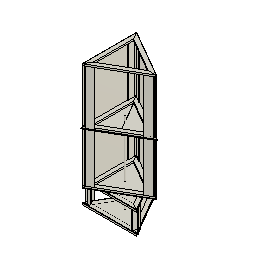
Periaktos (Autodesk Fusion 360 design; units mm, degrees)
Autodesk Fusion 360 part; units mm, degrees
sketch "Triangle" plane through (0, 0, 0) normal (0, 0, 1) x (1, 0, 0)
  line L0 (-609.6, -351.9527) -> (-609.6, -356.9527)
  line L1 (455.6207, -263.0527) -> (0, 526.1054)
  line L2 (0, 703.9054) -> (0, 526.1054)
  line L3 (0, -351.9527) -> (0, 703.9054)
  line L4 (-609.6, -351.9527) -> (-613.9301, -349.4527)
  line L5 (0, 703.9054) -> (-4.3301, 706.4054)
  line L6 (609.6, -351.9527) -> (613.9301, -349.4527)
  line L7 (0, 703.9054) -> (4.3301, 706.4054)
  line L8 (455.6207, -263.0527) -> (0, 0) construction
  circle A0 centre (0, 0) radius 11.1125
  line L9 (-609.6, -351.9527) -> (-455.6207, -263.0527)
  line L10 (609.6, -351.9527) -> (0, 703.9054)
  line L11 (0, 526.1054) -> (0, 0) construction
  line L12 (613.9301, -349.4527) -> (4.3301, 706.4054)
  line L13 (-609.6, -351.9527) -> (609.6, -351.9527)
  line L14 (-455.6207, -263.0527) -> (455.6207, -263.0527)
  line L15 (-4.3301, 706.4054) -> (-613.9301, -349.4527)
  line L16 (-609.6, -356.9527) -> (609.6, -356.9527)
  line L17 (609.6, -351.9527) -> (455.6207, -263.0527)
  line L18 (609.6, -351.9527) -> (609.6, -356.9527)
  line L19 (0, 703.9054) -> (-609.6, -351.9527)
  line L20 (-455.6207, -263.0527) -> (0, 0) construction
  line L21 (0, 526.1054) -> (-455.6207, -263.0527)
  line L22 (-609.6, -351.9527) -> (-558.8, -351.9527) construction
  point P0 (0, -263.0527)
  dimension "d82" = 88.9
  dimension "d83" = 88.9
  dimension "d84" = 88.9
  dimension "d85" = 5
  dimension "d86" = 5
  dimension "d87" = 5
  dimension "d88" = 1219.2
  dimension "d89" = 22.225
  dimension "d108" = 50.8
  constraint perpendicular L5 L15
  constraint perpendicular L7 L12
  constraint perpendicular L0 L16
  constraint perpendicular L4 L15
  constraint perpendicular L6 L12
  constraint perpendicular L16 L18
  constraint horizontal L13
  constraint coincident L8.end A0.centre
  constraint equal L13 L19
  constraint equal L10 L13
  constraint equal L11 L20
  constraint equal L8 L11
  constraint midpoint L3.start L13
  constraint perpendicular L0 L22
  constraint midpoint L14 P0
  measures "d82" distance of L1 L10
  measures "d83" distance of L19 L21
  measures "d84" distance of L13 L14
  measures "d85" distance of L10 L12
  measures "d86" distance of L15 L19
  measures "d87" distance of L13 L16
  measures "d88" distance of L0.start L6.start
  measures "d89" diameter of A0
  measures "d108" distance of L0.start L22.end
sketch "Supports" plane through (0, 0, 0) normal (0, 0, 1) x (1, 0, 0) in component "Periaktos"
  line L0 (-609.6, -351.9527) -> (609.6, -351.9527) construction
  line L1 (0, 703.9054) -> (-609.6, -351.9527) construction
  line L2 (609.6, -351.9527) -> (0, 703.9054) construction
  line L3 (-558.8, -351.9527) -> (-406.4, -351.9527)
  line L4 (-406.4, -351.9527) -> (-406.4, -339.2527)
  line L5 (-406.4, -339.2527) -> (-558.8, -339.2527)
  line L6 (-558.8, -339.2527) -> (-558.8, -351.9527)
  line L7 (-609.6, -351.9527) -> (-584.2, -307.9586) construction
  line L8 (-584.2, -307.9586) -> (-573.2015, -314.3086)
  line L9 (-573.2015, -314.3086) -> (-497.0015, -182.3264)
  line L10 (-497.0015, -182.3264) -> (-508, -175.9764)
  line L11 (-508, -175.9764) -> (-584.2, -307.9586)
  line L12 (-609.6, -351.9527) -> (-558.8, -351.9527) construction
  line L13 (584.2, -307.9586) -> (508, -175.9764)
  line L14 (573.2015, -314.3086) -> (584.2, -307.9586)
  line L15 (497.0015, -182.3264) -> (573.2015, -314.3086)
  line L16 (508, -175.9764) -> (497.0015, -182.3264)
  line L17 (406.4, -351.9527) -> (558.8, -351.9527)
  line L18 (406.4, -339.2527) -> (406.4, -351.9527)
  line L19 (558.8, -339.2527) -> (406.4, -339.2527)
  line L20 (558.8, -351.9527) -> (558.8, -339.2527)
  line L21 (-25.4, 659.9114) -> (-101.6, 527.9291)
  line L22 (-14.4015, 653.5614) -> (-25.4, 659.9114)
  line L23 (-90.6015, 521.5791) -> (-14.4015, 653.5614)
  line L24 (-101.6, 527.9291) -> (-90.6015, 521.5791)
  line L25 (101.6, 527.9291) -> (25.4, 659.9114)
  line L26 (90.6015, 521.5791) -> (101.6, 527.9291)
  line L27 (14.4015, 653.5614) -> (90.6015, 521.5791)
  line L28 (25.4, 659.9114) -> (14.4015, 653.5614)
  dimension "d110" = 152.4
  dimension "d111" = 12.7
  dimension "d112" = 50.8
  dimension "d113" = 12.7
  dimension "d114" = 152.4
  dimension "d115" = 50.8
  dimension "d117" = 360
  constraint coincident L0.start L1.end
  constraint parallel L1 L7
  constraint perpendicular L8 L11
  constraint perpendicular L10 L11
  constraint parallel L9 L11
  constraint collinear L1 L11
  constraint collinear L0 L3
  constraint parallel L3 L5
  constraint perpendicular L3 L6
  constraint perpendicular L3 L4
  constraint perpendicular L6 L12
  measures "d110" distance of L3.start L3.end
  measures "d111" distance of L3.start L5.end
  measures "d112" distance of L0.start L7.end
  measures "d113" distance of L7.end L8.end
  measures "d114" distance of L7.end L10.end
  measures "d115" distance of L3.start L0.start
extrude "Extrude1" add sketch "Triangle" along normal blind 12.7 from surface at 622.3 contours L2 L3 L9 L19 L21 | L3 L9 L13 L14 | L3 A0 L14 L21 | L3 L13 L14 L17 | L1 L2 L3 L10 L17 | L1 L3 A0 L14 makes body 1 in component "Periaktos"
extrude "Extrude2" add sketch "Triangle" along normal blind 38.1 from surface at 635 separate body contours L3 L9 L13 L14 | L3 L13 L14 L17 makes body 2 in component "Periaktos"
extrude "Extrude3" add sketch "Triangle" along normal blind 38.1 from surface at 635 separate body contours L2 L3 L9 L19 L21 makes body 3 in component "Periaktos"
extrude "Extrude4" add sketch "Triangle" along normal blind 38.1 from surface at 635 separate body contours L1 L2 L3 L10 L17 makes body 4 in component "Periaktos"
move_face "OffsetFaces1" offset -1.5875 4 faces at (-406.4, -351.9527, 626.5333) (203.2, -351.9527, 626.5333) (-203.2, 351.9527, 630.7667) (203.2, 351.9527, 626.5333) on bodies 1 in component "Periaktos"
extrude "Extrude5" add sketch "Triangle" against normal blind 38.1 from surface at 1841.5 separate body contours L3 L9 L13 L14 | L3 L13 L14 L17 makes body 5 in component "Periaktos"
extrude "Extrude6" add sketch "Triangle" against normal blind 38.1 from surface at 1841.5 separate body contours L2 L3 L9 L19 L21 makes body 6 in component "Periaktos"
extrude "Extrude7" add sketch "Triangle" against normal blind 38.1 from surface at 1841.5 separate body contours L1 L2 L3 L10 L17 makes body 7 in component "Periaktos"
extrude "Extrude8" add sketch "Triangle" against normal blind 12.7 from surface at 1803.4 separate body contours L2 L3 L9 L19 L21 | L3 L9 L13 L14 | L3 A0 L14 L21 makes body 8 in component "Periaktos"
extrude "Extrude9" add sketch "Triangle" against normal blind 12.7 from surface at 1803.4 separate body contours L3 L13 L14 L17 | L1 L2 L3 L10 L17 | L1 L3 A0 L14 makes body 9 in component "Periaktos"
move_face "OffsetFaces2" offset 12.7 4 faces at (-406.4, -351.9527, 1799.1667) (-203.2, 351.9527, 1794.9333) (203.2, -351.9527, 1799.1667) (203.2, 351.9527, 1799.1667) on bodies 8 9 in component "Periaktos"
extrude "Extrude10" add sketch "Triangle" against normal blind 38.1 from surface at 3060.7 separate body contours L3 L9 L13 L14 | L3 L13 L14 L17 makes body 10 in component "Periaktos"
extrude "Extrude11" add sketch "Triangle" against normal blind 38.1 from surface at 3060.7 separate body contours L2 L3 L9 L19 L21 makes body 11 in component "Periaktos"
extrude "Extrude12" add sketch "Triangle" against normal blind 38.1 from surface at 3060.7 separate body contours L1 L2 L3 L10 L17 makes body 12 in component "Periaktos"
extrude "Extrude 13" cut sketch "Supports" along normal up to surface (2349.5 mm away) from surface at 673.1 contours L3 L4 L5 L6 | L17 L18 L19 L20 bodies 5 8 9 in component "Periaktos"
extrude "Extrude14" add sketch "Supports" along normal up to surface (2349.5 mm away) from surface at 673.1 separate body contours L3 L4 L5 L6 | L17 L18 L19 L20 makes body 13 at (-508, -351.9527, 1456.2667) makes body 14 at (508, -339.2527, 1456.2667) in component "Periaktos"
extrude "Extrude15" cut sketch "Supports" along normal up to surface (2349.5 mm away) from surface at 673.1 contours L8 L9 L10 L11 | L21 L22 L23 L24 bodies 6 8 in component "Periaktos"
extrude "Extrude16" add sketch "Supports" along normal up to surface (2349.5 mm away) from surface at 673.1 separate body contours L8 L9 L10 L11 | L21 L22 L23 L24 makes body 15 at (-50.8, 615.9173, 1456.2667) makes body 16 at (-533.4, -219.9705, 1456.2667) in component "Periaktos"
extrude "Extrude17" cut sketch "Supports" along normal up to surface (2349.5 mm away) from surface at 673.1 contours L13 L14 L15 L16 | L25 L26 L27 L28 bodies 7 9 in component "Periaktos"
extrude "Extrude18" add sketch "Supports" along normal up to surface (2349.5 mm away) from surface at 673.1 separate body contours L13 L14 L15 L16 | L25 L26 L27 L28 makes body 17 at (558.8, -263.9645, 1456.2667) makes body 18 at (39.8015, 609.5673, 1456.2667) in component "Periaktos"
extrude "Extrude19" add sketch "Triangle" along normal up to surface (2438.4 mm away) from surface at 622.3 separate body contours L0 L13 L16 L18 makes body 19 in component "Periaktos"
extrude "Extrude20" add sketch "Triangle" along normal up to surface (2438.4 mm away) from surface at 622.3 separate body contours L4 L5 L15 L19 makes body 20 in component "Periaktos"
extrude "Extrude21" add sketch "Triangle" along normal up to surface (2438.4 mm away) from surface at 622.3 separate body contours L6 L7 L10 L12 makes body 21 in component "Periaktos"
sketch "Supports (2)" plane through (0, 0, 0) normal (0, 0, 1) x (1, 0, 0) in component "Pedestal"
  line L0 (-455.6207, -263.0527) -> (455.6207, -263.0527) construction
  line L1 (0, 526.1054) -> (-455.6207, -263.0527) construction
  line L2 (455.6207, -263.0527) -> (0, 526.1054) construction
  line L3 (-609.6, -351.9527) -> (609.6, -351.9527) construction
  line L4 (0, 703.9054) -> (-609.6, -351.9527) construction
  line L5 (609.6, -351.9527) -> (0, 703.9054) construction
  line L6 (-609.6, -351.9527) -> (-455.6207, -263.0527) construction
  line L7 (0, 703.9054) -> (0, 526.1054) construction
  line L8 (609.6, -351.9527) -> (455.6207, -263.0527) construction
  circle A0 centre (0, 0) radius 10.668
  line L9 (-609.6, -351.9527) -> (-584.2, -307.9586) construction
  line L10 (-584.2, -307.9586) -> (-508, -175.9764)
  line L11 (-508, -175.9764) -> (-518.9985, -169.6264)
  line L12 (-518.9985, -169.6264) -> (-595.1985, -301.6086)
  line L13 (-595.1985, -301.6086) -> (-584.2, -307.9586)
  line L14 (0, 703.9054) -> (-25.4, 659.9114) construction
  line L15 (-25.4, 659.9114) -> (-36.3985, 666.2614)
  line L16 (-36.3985, 666.2614) -> (-112.5985, 534.2791)
  line L17 (-112.5985, 534.2791) -> (-101.6, 527.9291)
  line L18 (-101.6, 527.9291) -> (-25.4, 659.9114)
  line L19 (25.4, 659.9114) -> (101.6, 527.9291)
  line L20 (36.3985, 666.2614) -> (25.4, 659.9114)
  line L21 (112.5985, 534.2791) -> (36.3985, 666.2614)
  line L22 (101.6, 527.9291) -> (112.5985, 534.2791)
  line L23 (508, -175.9764) -> (584.2, -307.9586)
  line L24 (518.9985, -169.6264) -> (508, -175.9764)
  line L25 (595.1985, -301.6086) -> (518.9985, -169.6264)
  line L26 (584.2, -307.9586) -> (595.1985, -301.6086)
  line L27 (-44.45, 602.3054) -> (44.45, 602.3054)
  line L28 (44.45, 602.3054) -> (44.45, 564.2054)
  line L29 (44.45, 564.2054) -> (-44.45, 564.2054)
  line L30 (-44.45, 564.2054) -> (-44.45, 602.3054)
  line L31 (0, 703.9054) -> (0, 602.3054) construction
  line L32 (-510.8413, -243.6079) -> (-466.3913, -320.5976)
  line L33 (-466.3913, -320.5976) -> (-499.3868, -339.6476)
  line L34 (-499.3868, -339.6476) -> (-543.8368, -262.6579)
  line L35 (-543.8368, -262.6579) -> (-510.8413, -243.6079)
  line L36 (466.3913, -320.5976) -> (510.8413, -243.6079)
  line L37 (510.8413, -243.6079) -> (543.8368, -262.6579)
  line L38 (543.8368, -262.6579) -> (499.3868, -339.6476)
  line L39 (499.3868, -339.6476) -> (466.3913, -320.5976)
  dimension "d156" = 21.336
  dimension "d157" = 50.8
  dimension "d158" = 152.4
  dimension "d159" = 12.7
  dimension "d162" = 50.8
  dimension "d163" = 12.7
  dimension "d164" = 152.4
  dimension "d168" = 360
  dimension "d181" = 88.9
  dimension "d182" = 38.1
  dimension "d183" = 101.6
  dimension "d185" = 360
  constraint coincident A0.centre origin
  constraint coincident L3.start L4.end
  constraint coincident L4 L9.end
  constraint perpendicular L10 L13
  constraint perpendicular L10 L11
  constraint parallel L10 L12
  constraint collinear L4 L10
  constraint coincident L4.start L5.end
  constraint parallel L4 L14
  constraint perpendicular L15 L18
  constraint perpendicular L17 L18
  constraint parallel L16 L18
  constraint collinear L4 L18
  constraint horizontal L27
  constraint vertical L28
  constraint horizontal L29
  constraint vertical L30
  constraint midpoint L27 L31.end
  constraint vertical L31
  measures "d156" diameter of A0
  measures "d157" distance of L3.start L9.end
  measures "d158" distance of L9.end L10.end
  measures "d159" distance of L9.end L12.end
  measures "d162" distance of L4.start L14.end
  measures "d163" distance of L14.end L15.end
  measures "d164" distance of L14.end L17.end
  measures "d181" distance of L27.start L27.end
  measures "d182" distance of L27.start L29.end
  measures "d183" distance of L4.start L31.end
extrude "Extrude1'" add sketch "Triangle" along normal blind 38.1 from surface at 38.1 separate body contours L3 L9 L13 L14 | L3 L13 L14 L17 makes body 22 in component "Pedestal"
extrude "Extrude2'" add sketch "Triangle" along normal blind 38.1 from surface at 38.1 separate body contours L2 L3 L9 L19 L21 makes body 23 in component "Pedestal"
extrude "Extrude3'" add sketch "Triangle" along normal blind 38.1 from surface at 38.1 separate body contours L1 L2 L3 L10 L17 makes body 24 in component "Pedestal"
extrude "Extrude4'" add sketch "Triangle" along normal blind 12.7 from surface at 76.2 separate body contours L2 L3 L9 L19 L21 | L3 L9 L13 L14 | L3 A0 L14 L21 | L3 L13 L14 L17 | L1 L2 L3 L10 L17 | L1 L3 A0 L14 | L3 A0 | L3 A0 makes body 25 in component "Pedestal"
extrude "Extrude5'" add sketch "Triangle" against normal blind 12.7 from surface at 558.8 separate body contours L2 L3 L9 L19 L21 | L3 L9 L13 L14 | L3 A0 L14 L21 | L3 L13 L14 L17 | L1 L2 L3 L10 L17 | L1 L3 A0 L14 makes body 26 in component "Pedestal"
extrude "Extrude6'" add sketch "Triangle" against normal blind 38.1 from surface at 546.1 separate body contours L3 L9 L13 L14 | L3 L13 L14 L17 makes body 27 in component "Pedestal"
extrude "Extrude7'" add sketch "Triangle" against normal blind 38.1 from surface at 546.1 separate body contours L2 L3 L9 L19 L21 makes body 28 in component "Pedestal"
extrude "Extrude8'" add sketch "Triangle" against normal blind 38.1 from surface at 546.1 separate body contours L1 L2 L3 L10 L17 makes body 29 in component "Pedestal"
extrude "Extrude9'" add sketch "Supports (2)" along normal up to surface (419.1 mm away) from surface at 88.9 separate body contours L32 L33 L34 L35 makes body 30 in component "Pedestal"
extrude "Extrude10'" add sketch "Supports (2)" along normal up to surface (419.1 mm away) from surface at 88.9 separate body contours L27 L28 L29 L30 makes body 31 in component "Pedestal"
extrude "Extrude11'" add sketch "Supports (2)" along normal up to surface (419.1 mm away) from surface at 88.9 separate body contours L36 L37 L38 L39 makes body 32 in component "Pedestal"
extrude "Extrude12'" add sketch "Supports (2)" along normal up to surface (508 mm away) from surface at 38.1 separate body contours L10 L11 L12 L13 | L15 L16 L17 L18 makes body 33 at (-61.7985, 622.2673, 207.4333) makes body 34 at (-544.3985, -213.6205, 207.4333) in component "Pedestal"
extrude "Extrude13" add sketch "Supports (2)" along normal up to surface (508 mm away) from surface at 38.1 separate body contours L19 L20 L21 L22 | L23 L24 L25 L26 makes body 35 at (569.7985, -257.6145, 207.4333) makes body 36 at (87.1985, 578.2732, 207.4333) in component "Pedestal"
extrude "Extrude14'" add sketch "Supports (2)" along normal blind 1828.8 from surface at 88.9 separate body contours A0 makes body 37 in component "Pedestal"
component "Periaktos" placed x (0.866025, 0.5, 0) y (-0.5, 0.866025, 0) z (0, 0, 1) at (0, 0, 0)
component "Pedestal" placed x (1, 0, 0) y (0, 1, 0) z (0, 0, 1) at (0, 0, 0)
hidden bodies 19
equation "d65 = ( -1 / 16 ) * 1 in"
equation "d89 = ( 7 / 8 ) * 1 in"
named bodies: "Bottom Triangle Edge C", "Bottom Triangle Edge B", "Bottom Triangle Edge A", "Bottom Triangle OSB", "Triangle Left OSB", "Triangle Right OSB", "Middle Triangle Edge A", "Middle Triangle Edge B", "Middle Triangle Edge C", "Top Triangle Edge A", "Top Triangle Edge B", "Top Triangle Edge C", "Support Edge A Left", "Support Edge A Right", "Support Edge B Left", "Support Edge B Right", "Support Edge C Left", "Support Edge C Right", "Panel A", "Panel B", "Panel C", "Top Triangle OSB", "Corner Leg AB", "Corner Leg BC", "Corner Leg AC", "Pipe"
